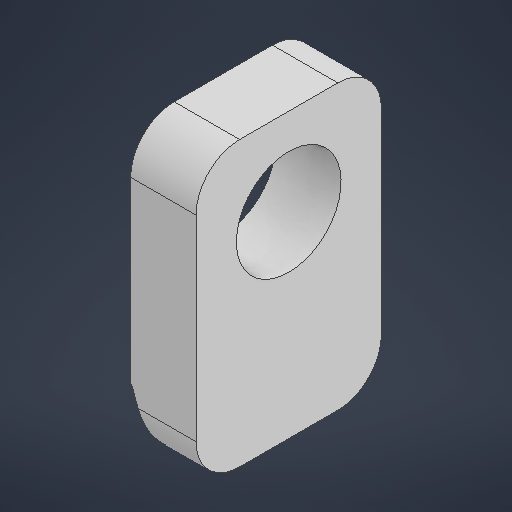
# Autodesk Inventor part: P_PIN
Saved by Autodesk Inventor 2026.2 (Build 302298000, 298)
## iProperties
Created: 2026-02-27
Part Number: P_PIN
Material: Generisch
Document SubType Name: Modeling
Designer: FAL
Density: 1 g/cm^3
Appearance: Vorgabe
Author: FAL
Autodesk Inventor part; units mm, degrees
ref_plane "YZ Plane" through (0, 0, 0) normal (1, 0, 0) x (0, 1, 0)
ref_plane "XZ Plane" through (0, 0, 0) normal (0, 1, 0) x (-1, 0, 0)
ref_plane "XY Plane" through (0, 0, 0) normal (0, 0, 1) x (1, 0, 0)
sketch "Skizze1" plane through (0, 0, 0) normal (1, 0, 0) x (0, 1, 0)
  line L0 (-4.25, -6.5) -> (4.25, -6.5)
  line L1 (4.25, -6.5) -> (4.25, 6.5)
  line L2 (4.25, 6.5) -> (-4.25, 6.5)
  line L3 (-4.25, 6.5) -> (-4.25, -6.5)
  line L4 (-4.25, -6.5) -> (4.25, 6.5) construction
  line L5 (4.25, -6.5) -> (-4.25, 6.5) construction
  point P0 (0, 0)
  dimension "d0" = 8.5
  dimension "d1" = 13
  constraints: 12 end point, 2 midpoint, 2 parallel, 1 horizontal, 1 perpendicular
  measures "d0" distance between parallel lines of L3 L1
  measures "d1" distance between parallel lines of L0 L2
extrude "Extrusion1" add sketch "Skizze1" along normal blind 3
sketch "Skizze3" plane through (0, 0, 0) normal (0, 1, 0) x (-1, 0, 0)
  line L0 (-1.0667, -6.5) -> (-0.0476, -3.7)
  line L1 (-0.0476, -3.7) -> (3.1717, -7.0921)
  line L2 (3.1717, -7.0921) -> (1.0847, -12.4156)
  line L3 (1.0847, -12.4156) -> (-1.0667, -6.5)
  line L4 (0, -6.5) -> (-3, -6.5) projected
  line L5 (0, -6.5) -> (0, 6.5) projected
  point P0 (0, 0)
  dimension "d11" = 2.8
  dimension "d12" = 20
  constraints: 8 end point, 1 point on line, 1 other
  measures "d11" distance from line of L4 L0.end
  measures "d12" angle to the sketch y axis of L0
extrude "Extrusion3" cut sketch "Skizze3" along normal mid plane 10.75
fillet "Rundung1" radius 2 4 edges at (1.5, 4.25, 6.5) (1.5, -4.25, 6.5) (2.0334, 4.25, -6.5) (2.0334, -4.25, -6.5)
sketch "Skizze2" plane through (0, 0, 0) normal (-1, 0, 0) x (0, 0, 1)
  circle A0 centre (2.5, 0) radius 2.4
  line L0 (6.5, 2.25) -> (6.5, -2.25) projected
  point P0 (0, 0)
  dimension "d6" = 4.8
  dimension "d13" = 4
  constraints: 1 centre point, 1 horizontal alignment
  measures "d6" diameter of A0
  measures "d13" distance from line of L0 A0.centre
extrude "Extrusion2" cut sketch "Skizze2" against normal blind 10.75
